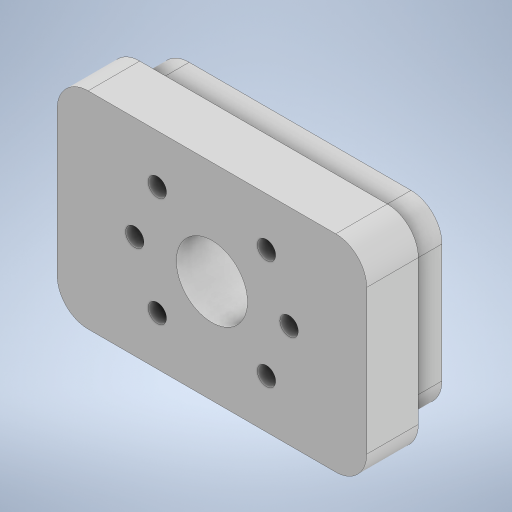
# Autodesk Inventor part: 2x3_Spacer_Rear_metal
Saved by Autodesk Inventor 2023 (Build 270158000, 158)
## iProperties
Created: 2022-05-03
Part Number: 2x3_Spacer_Rear_metal
Material: Generic
Document SubType Name: Modeling
Designer: plebbb
Density: 1 g/cm^3
Appearance: Default
Mass: 109.593 g
Surface Area: 204.871 cm^2
Volume: 109.593 cm^3
Author: plebbb
Autodesk Inventor part; units mm, degrees
ref_plane "YZ Plane" through (0, 0, 0) normal (1, 0, 0) x (0, 1, 0)
ref_plane "XZ Plane" through (0, 0, 0) normal (0, 1, 0) x (-1, 0, 0)
sketch "Sketch1" plane through (0, 0, 0) normal (0, 0, 1) x (1, 0, 0)
  line L0 (7.62, 0) -> (62.23, 0)
  line L1 (69.85, 7.62) -> (69.85, 36.83)
  line L2 (62.23, 44.45) -> (7.62, 44.45)
  line L3 (0, 36.83) -> (0, 7.62)
  arc A0 (7.62, 44.45) -> (0, 36.83) centre (7.62, 36.83) ccw
  arc A1 (0, 7.62) -> (7.62, 0) centre (7.62, 7.62) ccw
  arc A2 (62.23, 0) -> (69.85, 7.62) centre (62.23, 7.62) ccw
  arc A3 (69.85, 36.83) -> (62.23, 44.45) centre (62.23, 36.83) ccw
  point P0 (0, 0)
  point P1 (69.85, 44.45)
  point P2 (69.85, 0)
  point P3 (0, 44.45)
  dimension "d0" = 69.85
  dimension "d1" = 44.45
  dimension "d2" = 7.62
  constraints: 8 end point, 8 point on circle, 8 point on line, 8 tangent, 4 centre point, 3 equal radius, 2 parallel, 1 horizontal, 1 perpendicular
  measures "d0" distance of point (69.85, 44.45) point (0, 44.45)
  measures "d1" distance of point (69.85, 0) point (69.85, 44.45)
  measures "d2" radius of A0
extrude "Extrusion1" add sketch "Sketch1" along normal blind 9
sketch "Sketch2" plane through (0, 0, 9) normal (0, 0, 1) x (1, 0, 0)
  line L0 (4.445, -3.175) -> (65.405, -3.175)
  line L1 (73.025, 4.445) -> (73.025, 40.005)
  line L2 (65.405, 47.625) -> (4.445, 47.625)
  line L3 (-3.175, 40.005) -> (-3.175, 4.445)
  arc A0 (4.445, 47.625) -> (-3.175, 40.005) centre (4.445, 40.005) ccw
  arc A1 (-3.175, 4.445) -> (4.445, -3.175) centre (4.445, 4.445) ccw
  arc A2 (65.405, -3.175) -> (73.025, 4.445) centre (65.405, 4.445) ccw
  arc A3 (73.025, 40.005) -> (65.405, 47.625) centre (65.405, 40.005) ccw
  line L4 (62.23, 44.45) -> (7.62, 44.45) construction
  line L5 (0, 36.83) -> (0, 7.62) construction
  point P0 (0, 0)
  point P1 (73.025, 47.625)
  point P2 (73.025, -3.175)
  point P3 (-3.175, 47.625)
  point P4 (34.925, 47.625)
  point P5 (34.925, 44.45)
  point P6 (-3.175, 22.225)
  point P7 (0, 22.225)
  dimension "d5" = 76.2
  dimension "d6" = 50.8
  dimension "d7" = 7.62
  constraints: 8 end point, 8 point on circle, 8 tangent, 6 point on line, 4 centre point, 4 midpoint, 3 equal radius, 2 parallel, 1 horizontal, 1 horizontal alignment, 1 perpendicular, 1 vertical alignment
  measures "d5" distance of point (73.025, 47.625) point (-3.175, 47.625)
  measures "d6" distance of point (73.025, -3.175) point (73.025, 47.625)
  measures "d7" radius of A0
extrude "Extrusion2" add sketch "Sketch2" along normal blind 12.7
fillet "Fillet1" [suppressed]
sketch "Sketch3" plane through (0, 0, 21.7) normal (0, 0, 1) x (1, 0, 0)
  line L0 (65.405, 47.625) -> (4.445, 47.625) construction
  line L1 (65.405, 47.625) -> (4.445, 47.625) construction
  line L2 (-3.175, 40.005) -> (-3.175, 4.445) construction
  line L3 (-3.175, 40.005) -> (-3.175, 4.445) construction
  circle A0 centre (34.925, 22.225) radius 8.75
  circle A1 centre (34.925, 22.225) radius 19 construction
  circle A2 centre (21.49, 35.66) radius 2.25
  circle A3 centre (48.36, 35.66) radius 2.25
  circle A4 centre (15.925, 22.225) radius 2.25
  circle A5 centre (53.925, 22.225) radius 2.25
  circle A6 centre (21.49, 8.79) radius 2.25
  circle A7 centre (48.36, 8.79) radius 2.25
  line L4 (21.49, 35.66) -> (34.925, 22.225) construction
  line L5 (34.925, 22.225) -> (15.925, 22.225) construction
  point P0 (0, 0)
  point P1 (34.925, 47.625)
  point P2 (-3.175, 22.225)
  point P3 (-3.175, 22.225)
  dimension "d11" = 17.5
  dimension "d14" = 4.5
  dimension "d15" = 38
  dimension "d16" = 45
  constraints: 8 centre point, 6 point on circle, 5 equal radius, 5 horizontal alignment, 4 end point, 3 midpoint, 3 vertical alignment, 1 coincident
  measures "d11" diameter of A0
  measures "d14" diameter of A2
  measures "d15" diameter of A1
  measures "d16" angle of L5 L4
extrude "Extrusion3" cut sketch "Sketch3" against normal up to surface (21.7 mm away)
chamfer "Chamfer1" distance 1.27 angle 45 6 edges at (46.11, 35.66, 0) (19.24, 35.66, 0) (13.675, 22.225, 0) (51.675, 22.225, 0) (46.11, 8.79, 0) (19.24, 8.79, 0)
sketch "Sketch4" plane through (7.62, 0, 0) normal (0, -1, 0) x (1, 0, 0)
  point P0 (-7.62, 0)
ref_plane "Work Plane1" through (-0.635, 46.99, -50.8) normal (0, 1, 0) x (0, 0, 1)
sketch "Sketch8" plane through (0, 0, 0) normal (0, 0, -1) x (-1, 0, 0)
  point P0 (0, 0)
fillet "Fillet2" radius 0.635 1 edges at (26.175, 22.225, 0)
body "Solid1"
